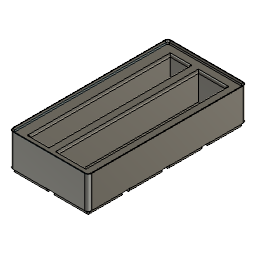
powerBank_double_2x4 (Autodesk Fusion 360 design; units mm, degrees)
part number: 2026-05-20-20-07-00-242
Autodesk Fusion 360 part; units mm, degrees
ref_plane "WorkPlane1" through (0, 0, 0) normal (0, 0, 1) x (1, 0, 0)
sketch "Base plate sketch" plane through (0, 0, 0) normal (0, 0, 1) x (1, 0, 0)
  line L0 (-0.25, -0.25) -> (41.75, -0.25)
  line L1 (41.75, -0.25) -> (41.75, 41.75)
  line L2 (41.75, 41.75) -> (-0.25, 41.75)
  line L3 (-0.25, 41.75) -> (-0.25, -0.25)
  dimension "d2" = 0.25
  dimension "d3" = 0.25
  dimension "d4" = 42
  dimension "d5" = 42
  constraint horizontal L0
  constraint vertical L1
  constraint horizontal L2
  constraint vertical L3
  measures "d2" vertical distance of origin L0.start
  measures "d3" horizontal distance of origin L2.end
  measures "d4" horizontal distance of L0.start L0.end
  measures "d5" vertical distance of L0.end L1.end
extrude "Base top section extrude" add sketch "Base plate sketch" against normal blind 2.4 makes body 1
fillet "Base corner fillet" radius 4 8 edges at (-0.25, -0.25, -1.2) (41.75, -0.25, -1.2) (41.75, -0.25, -1.2) (41.75, 41.75, -1.2) (41.75, 41.75, -1.2) (-0.25, 41.75, -1.2) (-0.25, 41.75, -1.2) (-0.25, -0.25, -1.2) on bodies 1
chamfer "Chamfer1" distance 2.4 angle 45 8 edges at (0.9216, 40.5784, -2.4) (-0.25, 20.75, -2.4) (0.9216, 0.9216, -2.4) (20.75, -0.25, -2.4) (40.5784, 0.9216, -2.4) (41.75, 20.75, -2.4) (40.5784, 40.5784, -2.4) (20.75, 41.75, -2.4) on bodies 1
extrude "Extrude2" add 1 faces at (15.6168, 15.0833, -2.4) along direction (0, 0, -1) blind 2.6 on bodies 1 bodies 1
chamfer "Chamfer2" distance 0.8 angle 45 8 edges at (2.6186, 38.8814, -5) (20.75, 39.35, -5) (38.8814, 38.8814, -5) (39.35, 20.75, -5) (38.8814, 2.6186, -5) (20.75, 2.15, -5) (2.6186, 2.6186, -5) (2.15, 20.75, -5) on bodies 1
pattern_linear "R-Pattern1" count 2 spacing 42 along (1, 0, 0) count 4 spacing 42 along (0, 1, 0) of bodies 1 makes body 2 at (68.4167, 16.4167, 0) makes body 3 at (26.4167, 55.75, 0) makes body 4 at (54.4167, 55.75, 0) makes body 5 at (26.4167, 97.75, 0) makes body 6 at (54.4167, 97.75, 0) makes body 7 at (26.4167, 139.75, 0) makes body 8 at (69.75, 141.0833, 0)
sketch "Simple box sketch" plane through (0, 0, 0) normal (0, 0, 1) x (1, 0, 0)
  line L0 (0, 0) -> (83.5, 0)
  line L1 (83.5, 0) -> (83.5, 167.5)
  line L2 (83.5, 167.5) -> (0, 167.5)
  line L3 (0, 167.5) -> (0, 0)
  dimension "d18" = 83.5
  dimension "d19" = 167.5
  constraint horizontal L0
  constraint vertical L1
  constraint horizontal L2
  constraint vertical L3
  constraint coincident L0.start L3
  constraint coincident L3.end L0
  measures "d18" horizontal distance of L0.start L0.end
  measures "d19" vertical distance of L0.end L1.end
extrude "Simple box extrude" add sketch "Simple box sketch" along normal blind 30 separate body makes body 9
fillet "Bin body corner fillets" radius 3.75 8 edges at (83.5, 167.5, 15) (83.5, 0, 15) (83.5, 0, 15) (0, 0, 15) (0, 167.5, 15) (83.5, 167.5, 15) (0, 0, 15) (0, 167.5, 15) on bodies 9
ref_plane "WorkPlane2" through (0, 0, 30) normal (0, 0, 1) x (1, 0, 0)
sketch "Simple box at point sketch" plane through (0, 0, 30) normal (0, 0, 1) x (1, 0, 0)
  line L0 (0, 0) -> (83.5, 0)
  line L1 (83.5, 0) -> (83.5, 167.5)
  line L2 (83.5, 167.5) -> (0, 167.5)
  line L3 (0, 167.5) -> (0, 0)
  dimension "d25" = 83.5
  dimension "d26" = 167.5
  constraint horizontal L0
  constraint vertical L1
  constraint horizontal L2
  constraint vertical L3
  constraint coincident L0.start L3
  constraint coincident L3.end L0
  measures "d25" horizontal distance of L0.start L0.end
  measures "d26" vertical distance of L0.end L1.end
extrude "Simple box at point extrude" add sketch "Simple box at point sketch" along normal blind 4.4 separate body makes body 10
fillet "Lip body corner fillets" radius 3.75 8 edges at (83.5, 167.5, 32.2) (83.5, 0, 32.2) (0, 0, 32.2) (0, 167.5, 32.2) (83.5, 0, 32.2) (0, 0, 32.2) (0, 167.5, 32.2) (83.5, 167.5, 32.2) on bodies 10
ref_plane "WorkPlane3" through (0, 0, 35) normal (0, 0, 1) x (1, 0, 0)
sketch "Base plate sketch (1)" plane through (0, 0, 35) normal (0, 0, 1) x (1, 0, 0)
  line L0 (-0.5, -0.5) -> (84, -0.5)
  line L1 (84, -0.5) -> (84, 168)
  line L2 (84, 168) -> (-0.5, 168)
  line L3 (-0.5, 168) -> (-0.5, -0.5)
  dimension "d32" = 0.5
  dimension "d33" = 0.5
  dimension "d34" = 84.5
  dimension "d35" = 168.5
  constraint horizontal L0
  constraint vertical L1
  constraint horizontal L2
  constraint vertical L3
  measures "d32" vertical distance of origin L0.start
  measures "d33" horizontal distance of origin L2.end
  measures "d34" horizontal distance of L0.start L0.end
  measures "d35" vertical distance of L0.end L1.end
extrude "Base top section extrude (1)" add sketch "Base plate sketch (1)" against normal blind 2.4 separate body makes body 11
fillet "Base corner fillet (1)" radius 4.25 8 edges at (-0.5, -0.5, 33.8) (84, -0.5, 33.8) (84, -0.5, 33.8) (84, 168, 33.8) (84, 168, 33.8) (-0.5, 168, 33.8) (-0.5, 168, 33.8) (-0.5, -0.5, 33.8) on bodies 11
chamfer "Chamfer3" distance 2.4 angle 45 8 edges at (0.7448, 166.7552, 32.6) (-0.5, 83.75, 32.6) (0.7448, 0.7448, 32.6) (41.75, -0.5, 32.6) (82.7552, 0.7448, 32.6) (84, 83.75, 32.6) (82.7552, 166.7552, 32.6) (41.75, 168, 32.6) on bodies 11
extrude "Extrude6" add 1 faces at (28.4665, 110.4167, 32.6) along direction (0, 0, -1) blind 2.6 on bodies 11 bodies 11
ref_plane "WorkPlane4" through (41.75, 83.75, 34.4) normal (0, 0, 1) x (1, 0, 0)
sketch "Lip top chamfer" plane through (0, 0, 34.4) normal (0, 0, 1) x (1, 0, 0)
  line L0 (0, 0) -> (83.5, 0)
  line L1 (83.5, 0) -> (83.5, 167.5)
  line L2 (83.5, 167.5) -> (0, 167.5)
  line L3 (0, 167.5) -> (0, 0)
  dimension "d44" = 83.5
  dimension "d45" = 167.5
  constraint horizontal L0
  constraint vertical L1
  constraint horizontal L2
  constraint vertical L3
  constraint coincident L0.start L3
  constraint coincident L3.end L0
  measures "d44" horizontal distance of L0.start L0.end
  measures "d45" vertical distance of L0.end L1.end
extrude "Lip top chamfer cut" add sketch "Lip top chamfer" against normal blind 0.6 separate body makes body 12
combine "Combine1" operation cut target body 10 tool bodies 12 11
ref_plane "WorkPlane5" through (0, 0, 30) normal (0, 0, 1) x (1, 0, 0)
sketch "Simple box at point sketch (1)" plane through (0, 0, 30) normal (0, 0, 1) x (1, 0, 0)
  line L0 (1.2, 1.2) -> (82.3, 1.2)
  line L1 (82.3, 1.2) -> (82.3, 166.3)
  line L2 (82.3, 166.3) -> (1.2, 166.3)
  line L3 (1.2, 166.3) -> (1.2, 1.2)
  dimension "d49" = 1.2
  dimension "d50" = 1.2
  dimension "d51" = 81.1
  dimension "d52" = 165.1
  constraint horizontal L0
  constraint vertical L1
  constraint horizontal L2
  constraint vertical L3
  measures "d49" vertical distance of origin L0.start
  measures "d50" horizontal distance of origin L2.end
  measures "d51" horizontal distance of L0.start L0.end
  measures "d52" vertical distance of L0.end L1.end
extrude "Lip bottom chamfer extrude" add sketch "Simple box at point sketch (1)" along normal blind 2.55 separate body makes body 13
fillet "Fillet5" radius 2.55 8 edges at (1.2, 166.3, 31.275) (82.3, 166.3, 31.275) (82.3, 166.3, 31.275) (82.3, 1.2, 31.275) (82.3, 1.2, 31.275) (1.2, 1.2, 31.275) (1.2, 1.2, 31.275) (1.2, 166.3, 31.275) on bodies 13
chamfer "Chamfer4" distance 2.55 angle 45 8 edges at (1.9469, 1.9469, 32.55) (41.75, 1.2, 32.55) (81.5531, 1.9469, 32.55) (82.3, 83.75, 32.55) (81.5531, 165.5531, 32.55) (41.75, 166.3, 32.55) (1.9469, 165.5531, 32.55) (1.2, 83.75, 32.55) on bodies 13
combine "Combine2" operation cut target body 10 tool bodies 13
combine "Combine3" operation add target body 9 tool bodies 10
ref_plane "WorkPlane6" through (0, 0, 0) normal (0, 0, 1) x (1, 0, 0)
sketch "Base clearance cut sketch" plane through (0, 0, 0) normal (0, 0, 1) x (1, 0, 0)
  line L0 (3.75, 0) -> (79.75, 0)
  line L1 (83.5, 3.75) -> (83.5, 163.75)
  line L2 (79.75, 167.5) -> (3.75, 167.5)
  line L3 (0, 163.75) -> (0, 3.75)
  arc A0 (79.75, 0) -> (83.5, 3.75) centre (79.75, 3.75) ccw
  arc A1 (83.5, 163.75) -> (79.75, 167.5) centre (79.75, 163.75) ccw
  arc A2 (3.75, 167.5) -> (0, 163.75) centre (3.75, 163.75) ccw
  arc A3 (0, 3.75) -> (3.75, 0) centre (3.75, 3.75) ccw
  arc A4 (79.75, -10) -> (93.5, 3.75) centre (79.75, 3.75) ccw
  line L4 (93.5, 3.75) -> (93.5, 163.75)
  arc A5 (93.5, 163.75) -> (79.75, 177.5) centre (79.75, 163.75) ccw
  line L5 (79.75, 177.5) -> (3.75, 177.5)
  arc A6 (3.75, 177.5) -> (-10, 163.75) centre (3.75, 163.75) ccw
  line L6 (-10, 163.75) -> (-10, 3.75)
  arc A7 (-10, 3.75) -> (3.75, -10) centre (3.75, 3.75) ccw
  line L7 (3.75, -10) -> (79.75, -10)
  point P0 (83.5, 0)
  point P1 (83.5, 167.5)
  dimension "d59" = 83.5
  dimension "d60" = 167.5
  dimension "d61" = 3.75
  dimension "d62" = 10
  constraint horizontal L0
  constraint vertical L1
  constraint horizontal L2
  constraint vertical L3
  constraint coincident origin L3
  constraint coincident origin L0
  constraint coincident P0 L0
  constraint coincident P0 L1
  constraint tangent L0 A0
  constraint tangent L1 A0
  constraint coincident P1 L1
  constraint coincident P1 L2
  constraint tangent L1 A1
  constraint tangent L2 A1
  constraint tangent L2 A2
  constraint tangent L3 A2
  constraint tangent L3 A3
  constraint tangent L0 A3
  constraint equal A0 A1
  constraint equal A1 A2
  constraint equal A2 A3
  measures "d59" horizontal distance of origin P0
  measures "d60" vertical distance of P0 P1
  measures "d61" radius of A0
extrude "Base side clearance cut" cut sketch "Base clearance cut sketch" along normal blind 1000 and the other way blind 1000 bodies 1 2 3 4 5 6 7 8 9
combine "Combine4" operation add target body 9 tool bodies 2 3 4 5 6 7 8 1 1
sketch "Sketch8" plane through (0, 1.9, 0) normal (0, 1, 0) x (-1, 0, 0)
  line L0 (-79.75, 30.7) -> (-3.75, 30.7)
  line L1 (-3.75, 30.7) -> (-3.75, 32.6)
  line L2 (-3.75, 32.6) -> (-79.75, 32.6)
  line L3 (-79.75, 32.6) -> (-79.75, 30.7)
ref_plane "WorkPlane7" through (41.75, 83.75, 30) normal (0, 0, 1) x (1, 0, 0)
sketch "Sketch9" plane through (1.9, 0, 0) normal (1, 0, 0) x (0, 1, 0)
  line L0 (3.75, 30.7) -> (163.75, 30.7)
  line L1 (163.75, 30.7) -> (163.75, 32.6)
  line L2 (163.75, 32.6) -> (3.75, 32.6)
  line L3 (3.75, 32.6) -> (3.75, 30.7)
sketch "Sketch10" plane through (0, 0, 30) normal (0, 0, 1) x (1, 0, 0)
  line L0 (3.75, 1.9) -> (3.75, 10.2)
  line L1 (3.75, 10.2) -> (81.6, 10.2)
  line L2 (81.6, 10.2) -> (70.8, 10.2)
  line L3 (70.8, 10.2) -> (70.8, 157.2)
  line L4 (70.8, 157.2) -> (81.6, 157.2)
  line L5 (81.6, 157.2) -> (81.6, 10.2)
  line L6 (70.8, 10.2) -> (42.7, 10.2)
  line L7 (42.7, 10.2) -> (42.7, 157.2)
  line L8 (42.7, 157.2) -> (70.8, 157.2)
  line L9 (70.8, 157.2) -> (70.8, 10.2)
  line L10 (42.7, 10.2) -> (31.9, 10.2)
  line L11 (31.9, 10.2) -> (31.9, 157.2)
  line L12 (31.9, 157.2) -> (42.7, 157.2)
  line L13 (42.7, 157.2) -> (42.7, 10.2)
  line L14 (31.9, 10.2) -> (12.9, 10.2)
  line L15 (12.9, 10.2) -> (12.9, 157.2)
  line L16 (12.9, 157.2) -> (31.9, 157.2)
  line L17 (31.9, 157.2) -> (31.9, 10.2)
  dimension "d68" = 8.3
  dimension "d69" = 10.8
  dimension "d70" = 147
  dimension "d71" = 28.1
  dimension "d72" = 147
  dimension "d73" = 10.8
  dimension "d74" = 147
  dimension "d75" = 19
  dimension "d76" = 147
  constraint vertical L0
  constraint perpendicular L0 L1
  constraint horizontal L2
  constraint vertical L3
  constraint horizontal L4
  constraint vertical L5
  constraint horizontal L6
  constraint vertical L7
  constraint horizontal L8
  constraint vertical L9
  constraint horizontal L10
  constraint vertical L11
  constraint horizontal L12
  constraint vertical L13
  constraint horizontal L14
  constraint vertical L15
  constraint horizontal L16
  constraint vertical L17
  measures "d68" distance of L0.start L0.end
  measures "d69" distance of L1.end L2.end
  measures "d70" distance of L1.end L4.end
  measures "d71" distance of L2.end L6.end
  measures "d72" distance of L2.end L3.end
  measures "d73" distance of L6.end L10.end
  measures "d74" distance of L6.end L7.end
  measures "d75" distance of L10.end L14.end
  measures "d76" distance of L10.end L11.end
extrude "Extrude10" cut sketch "Sketch10" against normal blind 28 contours L1 L11 L14 L15 L16 L17 | L1 L3 L6 L7 L8 L9 L13 bodies 9
fillet "Fillet6" radius 2 4 edges at (12.9, 83.7, 30) (22.4, 10.2, 30) (56.75, 10.2, 30) (42.7, 83.7, 30) on bodies 9
fillet "Fillet7" radius 2 4 edges at (31.9, 82.7, 30) (70.8, 82.7, 30) (55.75, 157.2, 30) (21.4, 157.2, 30) on bodies 9
equation "d6 = -( 2.40 mm )"
equation "d36 = -( 2.40 mm )"
equation "d46 = -( 0.60 mm )"
named bodies: "Base", "Base (1)", "Base (2)", "Base (3)", "Base (4)", "Base (5)", "Base (6)", "Base (7)", "Gridfinity bin 4x2x5", "Lip body", "Lip cutout"
